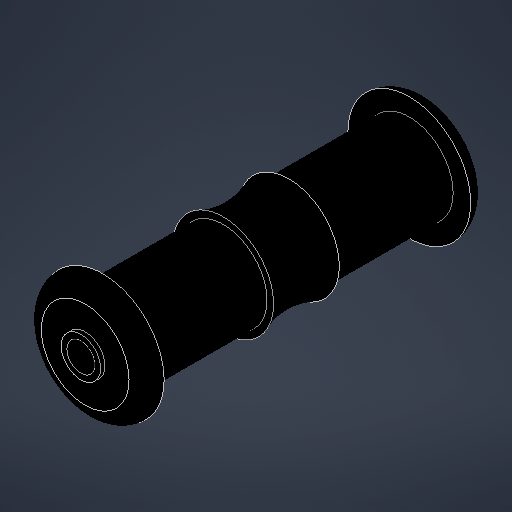
# Autodesk Inventor part: Dribbler Roller Seperator
Saved by Autodesk Inventor 2026.1 (Build 301233020, 233B)
## iProperties
Created: 2026-04-17
Part Number: Dribbler Roller Seperator
Material: Generic
Document SubType Name: Modeling
Designer: Bahaa
Mass: 3.05373 g
Surface Area: 21.2142 cm^2
Volume: 3.05373 cm^3
Density: 1 g/cm^3
Appearance: Black PLA
Author: Bahaa
Autodesk Inventor part; units mm, degrees
ref_plane "YZ Plane" through (0, 0, 0) normal (1, 0, 0) x (0, 1, 0)
ref_plane "XZ Plane" through (0, 0, 0) normal (0, 1, 0) x (-1, 0, 0)
ref_plane "XY Plane" through (0, 0, 0) normal (0, 0, 1) x (1, 0, 0)
sketch "Sketch1" plane through (0, 0, 0) normal (0, 1, 0) x (-1, 0, 0)
  circle A0 centre (0, 0) radius 1.5875
  circle A1 centre (0, 0) radius 2.25
  circle A2 centre (0, 0) radius 7
  circle A3 centre (0, 0) radius 5
  circle A4 centre (0, 0) radius 5.75
  dimension "d0" = 3.175
  dimension "d1" = 4.5
  dimension "d2" = 14
  dimension "d3" = 10
  dimension "d4" = 11.5
  constraints: 5 centre point, 5 coincident
  measures "d0" diameter of A0
  measures "d1" diameter of A1
  measures "d2" diameter of A2
  measures "d3" diameter of A3
  measures "d4" diameter of A4
extrude "Extrusion1" add sketch "Sketch1" against normal blind 0.5 contours A1
extrude "Extrusion2" add sketch "Sketch1" along normal blind 2 contours A1 | A2 | A3 | A4
extrude "Extrusion3" add sketch "Sketch1" along normal blind 13.75 from surface at 2 contours A1 | A3
extrude "Extrusion4" add sketch "Sketch1" along normal blind 3.75 from surface at 15.75 contours A1 | A3 | A4
fillet "Fillet1" radius 2 1 edges at (7, 0, 0)
mirror "Mirror1" about plane through (0, 19.5, 0) normal (0, 1, 0)
sketch "Sketch2" plane through (0, 0, 0) normal (1, 0, 0) x (0, 1, 0)
  line L0 (15.75, -5.75) -> (23.25, -5.75) projected
  line L1 (15.75, 5.75) -> (15.75, -5.75) projected
  arc A0 (23.25, -5.75) -> (15.75, -5.75) centre (19.5, -14.75) ccw
  line L2 (0, 0) -> (10, 0) construction
  point P0 (19.5, -5.75)
  point P1 (19.5, -5)
  dimension "d14" = 0.75
  dimension "d15" = 10
  constraints: 3 point on circle, 2 end point, 1 centre point, 1 horizontal, 1 midpoint, 1 point on line, 1 vertical alignment
  measures "d14" distance of point (19.5, -5.75) point (19.5, -5)
  measures "d15" distance of L2.start L2.end
revolve "Revolution1" cut sketch "Sketch2" angle 360 about axis through (0, 0, 0) along (0, 1, 0)
body "Solid1"
